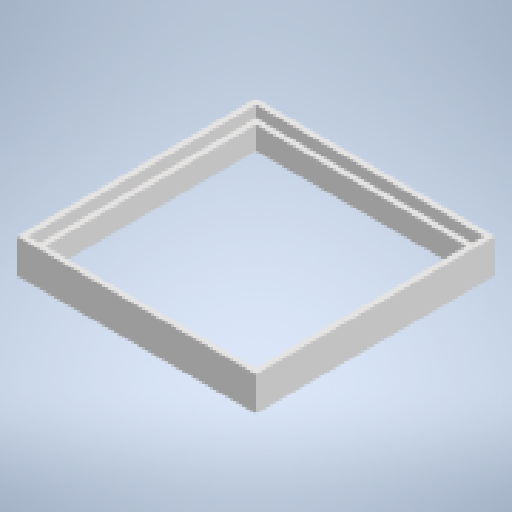
# Autodesk Inventor part: rebord2
Saved by Autodesk Inventor 2025.2 (Build 292293000, 293)
## iProperties
Created: 2025-02-20
Part Number: rebord2
Material: Générique
Document SubType Name: Modeling
Designer: antoi
Density: 1 g/cm^3
Appearance: Par défaut
Author: antoi
Autodesk Inventor part; units mm, degrees
ref_plane "YZ Plane" through (0, 0, 0) normal (1, 0, 0) x (0, 1, 0)
ref_plane "XZ Plane" through (0, 0, 0) normal (0, 1, 0) x (-1, 0, 0)
ref_plane "XY Plane" through (0, 0, 0) normal (0, 0, 1) x (1, 0, 0)
sketch "Esquisse2" plane through (0, 0, 0) normal (0, 1, 0) x (-1, 0, 0)
  line L0 (0, 0) -> (105, 0)
  line L1 (105, 0) -> (105, -105)
  line L2 (105, -105) -> (0, -105)
  line L3 (0, -105) -> (0, 0)
  line L4 (5, -5) -> (100, -5)
  line L5 (100, -5) -> (100, -100)
  line L6 (100, -100) -> (5, -100)
  line L7 (5, -100) -> (5, -5)
  dimension "d5" = 105
  dimension "d6" = 105
  dimension "d7" = 95
  dimension "d8" = 95
  constraints: 16 end point, 4 parallel, 2 horizontal, 2 perpendicular
  measures "d5" distance of L1.end L2.end
  measures "d6" distance of L0.end L1.end
  measures "d7" distance of L5.end L6.end
  measures "d8" distance of L4.end L5.end
extrude "Extrusion1" add sketch "Esquisse2" along normal blind 15
sketch "Esquisse3" plane through (0, 15, 0) normal (0, 1, 0) x (1, 0, 0)
  line L0 (-5, 5) -> (-100, 5) projected
  line L1 (-5, 5) -> (-100, 5)
  line L2 (-100, 5) -> (-100, 100)
  line L3 (-100, 100) -> (-5, 100)
  line L4 (-5, 100) -> (-5, 5)
  line L5 (-2.5, 2.5) -> (-102.5, 2.5)
  line L6 (-102.5, 2.5) -> (-102.5, 102.5)
  line L7 (-102.5, 102.5) -> (-2.5, 102.5)
  line L8 (-2.5, 102.5) -> (-2.5, 2.5)
  point P0 (0, 0)
  dimension "d11" = 95
  dimension "d12" = 95
  dimension "d13" = 100
  dimension "d14" = 100
  constraints: 16 end point, 4 parallel, 2 horizontal, 2 perpendicular
  measures "d11" distance of L2.end L3.end
  measures "d12" distance of L1.end L2.end
  measures "d13" distance of L6.end L7.end
  measures "d14" distance of L5.end L6.end
extrude "Extrusion2" cut sketch "Esquisse3" against normal blind 5
